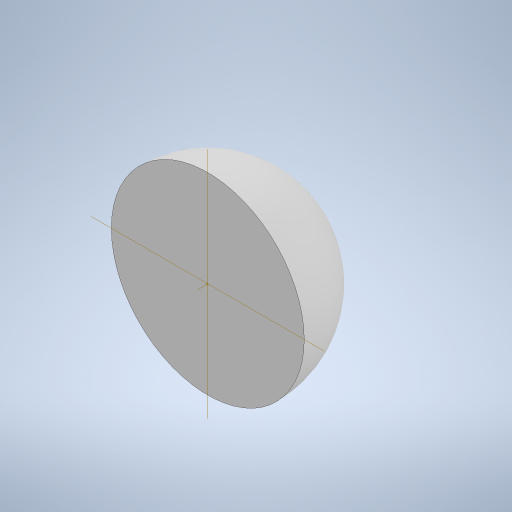
# Autodesk Inventor part: Hemisphere
Saved by Autodesk Inventor 2023.2 (Build 272271030, 271C)
## iProperties
Created: 2023-02-26
Part Number: Hemisphere
Material: Generisch
Document SubType Name: Modeling
Designer: mehan
Density: 1 g/cm^3
Appearance: Vorgabe
Author: mehan
Autodesk Inventor part; units mm, degrees
ref_plane "YZ Plane" through (0, 0, 0) normal (1, 0, 0) x (0, 1, 0)
ref_plane "XZ Plane" through (0, 0, 0) normal (0, 1, 0) x (-1, 0, 0)
ref_plane "XY Plane" through (0, 0, 0) normal (0, 0, 1) x (1, 0, 0)
sketch "Skizze1" plane through (0, 0, 0) normal (0, 0, 1) x (1, 0, 0)
  line L0 (-52.5, 0) -> (52.5, 0)
  arc A0 (52.5, 0) -> (-52.5, 0) centre (0, 0) ccw
  dimension "d2" = 105
  constraints: 2 end point, 2 point on circle, 1 centre point, 1 coincident, 1 horizontal
  measures "d2" distance of L0.end L0.start
revolve "Umdrehung1" add sketch "Skizze1" angle 180 about axis through (-52.5, 0, 0) along (-1, 0, 0)
